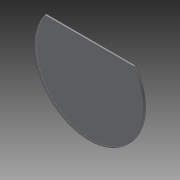
# Autodesk Inventor part: Mid Plate
Saved by Autodesk Inventor 2015 (Build 190159000, 159)
## iProperties
Created: 2014-11-13
Part Number: Mid Plate
Material: Generic
Document SubType Name: Modeling
Designer: karl
Density: 1 g/cm^3
Appearance: Default
Author: karl
Autodesk Inventor part; units mm, degrees
ref_plane "YZ Plane" through (0, 0, 0) normal (1, 0, 0) x (0, 1, 0)
ref_plane "XZ Plane" through (0, 0, 0) normal (0, 1, 0) x (-1, 0, 0)
ref_plane "XY Plane" through (0, 0, 0) normal (0, 0, 1) x (1, 0, 0)
sketch "Sketch1" plane through (0, 0, 0) normal (0, 1, 0) x (-1, 0, 0)
  circle A0 centre (0, 0) radius 90
  line L0 (73.4575, 52) -> (-73.4575, 52)
  dimension "d0" = 180
  dimension "d1" = 52
  constraints: 2 end point, 2 point on circle, 1 centre point, 1 coincident, 1 horizontal
  measures "d0" diameter of A0
  measures "d1" distance from line of point (0, 0) L0
extrude "Extrusion1" add sketch "Sketch1" along normal blind 3 contours A0 L0 picked at (17.1608, -0.9679)
sketch "Sketch2" plane through (0, 3, 0) normal (0, 1, 0) x (1, 0, 0)
  line L0 (-73.4575, -52) -> (73.4575, -52) projected
  line L1 (57, -52) -> (90, -52)
  line L2 (90, -52) -> (90, 90)
  line L3 (90, 90) -> (57, 90)
  line L4 (57, 90) -> (57, -52)
  arc A0 (73.4575, -52) -> (-73.4575, -52) centre (0, 0) ccw projected
  dimension "d4" = 57
  constraints: 8 end point, 2 parallel, 2 tangent, 1 horizontal, 1 perpendicular, 1 point on line
  measures "d4" distance from line of point (0, 0) L4
extrude "Extrusion2" cut sketch "Sketch2" against normal blind 3 contours L4 A0 L0 | L4 L3 L2 A0 | A0 L2 L1 picked at (60.2055, 26.0552)
sketch "Sketch3" plane through (0, 3, 0) normal (0, 1, 0) x (1, 0, 0)
  line L0 (29, -46) -> (-29, -46)
  line L1 (-29, -46) -> (-29, 22)
  line L2 (-29, 22) -> (29, 22)
  line L3 (29, 22) -> (29, -46)
  line L4 (-73.4575, -52) -> (57, -52) projected
  point P0 (0, 0)
  dimension "d7" = 6
  dimension "d8" = 74
  dimension "d9" = 29
  dimension "d10" = 29
  constraints: 8 end point, 2 parallel, 1 horizontal, 1 perpendicular
  measures "d7" distance between parallel lines of L4 L0
  measures "d8" distance between parallel lines of L4 L2
  measures "d9" distance from line of point (0, 0) L1
  measures "d10" distance from line of L3 point (0, 0)
extrude "Extrusion3" cut sketch "Sketch3" against normal blind 3
mirror "Mirror1" about plane through (0, 0, 0) normal (1, 0, 0) of "Extrusion2"
sketch "Sketch4" plane through (0, 3, 0) normal (0, 1, 0) x (1, 0, 0)
  line L0 (57, 69.6491) -> (57, -52) projected
  line L1 (57, -37) -> (60, -37)
  line L2 (60, -37) -> (60, -17)
  line L3 (60, -17) -> (57, -17)
  line L4 (57, -17) -> (57, -37)
  line L5 (-57, -52) -> (57, -52) projected
  line L6 (57, 13) -> (60, 13)
  line L7 (60, 13) -> (60, 33)
  line L8 (60, 33) -> (57, 33)
  line L9 (57, 33) -> (57, 13)
  point P0 (0, 0)
  dimension "d13" = 3
  dimension "d14" = 20
  dimension "d15" = 15
  dimension "d16" = 3
  dimension "d17" = 20
  dimension "d18" = 30
  constraints: 16 end point, 4 parallel, 2 horizontal, 2 perpendicular, 2 point on line
  measures "d13" distance of L3.end L2.end
  measures "d14" distance of L2.end L1.end
  measures "d15" distance between parallel lines of L5 L1
  measures "d16" distance of L8.end L7.end
  measures "d17" distance of L7.end L6.end
  measures "d18" distance between parallel lines of L3 L6
extrude "Extrusion4" add sketch "Sketch4" against normal blind 3
sketch "Sketch5" plane through (0, 3, 0) normal (0, 1, 0) x (1, 0, 0)
  line L0 (38, 53) -> (35, 53)
  line L1 (35, 53) -> (35, 43)
  line L2 (35, 43) -> (38, 43)
  line L3 (38, 43) -> (38, 53)
  line L4 (38, -42) -> (35, -42)
  line L5 (35, -42) -> (35, -32)
  line L6 (35, -32) -> (38, -32)
  line L7 (38, -32) -> (38, -42)
  line L8 (38, 8) -> (35, 8)
  line L9 (35, 8) -> (35, -12)
  line L10 (35, -12) -> (38, -12)
  line L11 (38, -12) -> (38, 8)
  line L12 (-57, -52) -> (57, -52) projected
  point P0 (0, 0)
  dimension "d21" = 3
  dimension "d22" = 10
  dimension "d23" = 3
  dimension "d24" = 10
  dimension "d25" = 3
  dimension "d26" = 20
  dimension "d27" = 10
  dimension "d28" = 20
  dimension "d29" = 35
  dimension "d30" = 35
  constraints: 24 end point, 6 parallel, 3 horizontal, 3 perpendicular, 2 point on line
  measures "d21" distance of L2.end L1.end
  measures "d22" distance of L1.end L0.end
  measures "d23" distance of L5.end L6.end
  measures "d24" distance of L4.end L5.end
  measures "d25" distance of L10.end L9.end
  measures "d26" distance of L9.end L8.end
  measures "d27" distance between parallel lines of L12 L4
  measures "d28" distance between parallel lines of L10 L6
  measures "d29" distance between parallel lines of L2 L8
  measures "d30" distance from line of point (0, 0) L5
extrude "Extrusion5" cut sketch "Sketch5" against normal blind 3
sketch "Sketch6" plane through (0, 3, 0) normal (0, 1, 0) x (1, 0, 0)
  line L0 (52.5, 31) -> (42.5, 31)
  line L1 (42.5, 31) -> (42.5, 28)
  line L2 (42.5, 28) -> (52.5, 28)
  line L3 (52.5, 28) -> (52.5, 31)
  line L4 (5, 31) -> (25, 31)
  line L5 (25, 31) -> (25, 28)
  line L6 (25, 28) -> (5, 28)
  line L7 (5, 28) -> (5, 31)
  line L8 (-57, -52) -> (57, -52) projected
  point P0 (0, 0)
  dimension "d33" = 10
  dimension "d34" = 3
  dimension "d35" = 20
  dimension "d36" = 3
  dimension "d37" = 5
  dimension "d38" = 17.5
  dimension "d39" = 80
  constraints: 16 end point, 4 parallel, 2 horizontal, 2 perpendicular, 1 point on line
  measures "d33" distance of L2.end L1.end
  measures "d34" distance of L1.end L0.end
  measures "d35" distance of L5.end L6.end
  measures "d36" distance of L4.end L5.end
  measures "d37" distance from line of point (0, 0) L7
  measures "d38" distance between parallel lines of L1 L5
  measures "d39" distance between parallel lines of L8 L6
extrude "Extrusion6" cut sketch "Sketch6" against normal blind 3
mirror "Mirror2" about plane through (0, 0, 0) normal (1, 0, 0) of "Extrusion4", "Extrusion5", "Extrusion6"
sketch "Sketch7" plane through (0, 3, 0) normal (0, 1, 0) x (1, 0, 0)
  line L0 (-1.75, 99) -> (1.75, 99)
  line L1 (1.75, 99) -> (1.75, 79)
  line L2 (1.75, 79) -> (-1.75, 79)
  line L3 (-1.75, 79) -> (-1.75, 99)
  point P0 (0, 0)
  point P1 (0, 79)
  dimension "d42" = 3.5
  dimension "d43" = 20
  dimension "d44" = 79
  constraints: 8 end point, 2 parallel, 1 horizontal, 1 midpoint, 1 perpendicular, 1 vertical alignment
  measures "d42" distance of L1.end L2.end
  measures "d43" distance of L0.end L1.end
  measures "d44" distance from line of point (0, 0) L2
extrude "Extrusion7" cut sketch "Sketch7" against normal blind 3
sketch "Sketch8" plane through (0, 3, 0) normal (0, 1, 0) x (1, 0, 0)
  line L0 (42.5, 14) -> (52.5, 14)
  line L1 (52.5, 14) -> (52.5, 11)
  line L2 (52.5, 11) -> (42.5, 11)
  line L3 (42.5, 11) -> (42.5, 14)
  line L4 (42.5, 28) -> (42.5, 31) projected
  line L5 (42.5, -37) -> (52.5, -37)
  line L6 (52.5, -37) -> (52.5, -34)
  line L7 (52.5, -34) -> (42.5, -34)
  line L8 (42.5, -34) -> (42.5, -37)
  line L9 (-57, -52) -> (57, -52) projected
  point P0 (0, 0)
  dimension "d47" = 10
  dimension "d48" = 3
  dimension "d49" = 10
  dimension "d50" = 3
  dimension "d51" = 45
  dimension "d52" = 15
  constraints: 16 end point, 4 parallel, 2 collinear, 2 horizontal, 2 perpendicular
  measures "d47" distance of L1.end L2.end
  measures "d48" distance of L0.end L1.end
  measures "d49" distance of L7.end L6.end
  measures "d50" distance of L6.end L5.end
  measures "d51" distance between parallel lines of L7 L2
  measures "d52" distance between parallel lines of L9 L5
extrude "Extrusion8" cut sketch "Sketch8" against normal blind 3
sketch "Sketch9" plane through (0, 3, 0) normal (0, 1, 0) x (1, 0, 0)
  line L0 (-57, -52) -> (57, -52) projected
  line L1 (50, -52) -> (30, -52)
  line L2 (30, -52) -> (30, -55)
  line L3 (30, -55) -> (50, -55)
  line L4 (50, -55) -> (50, -52)
  line L5 (20, -52) -> (10, -52)
  line L6 (10, -52) -> (10, -55)
  line L7 (10, -55) -> (20, -55)
  line L8 (20, -55) -> (20, -52)
  point P0 (0, 0)
  dimension "d55" = 20
  dimension "d56" = 3
  dimension "d57" = 10
  dimension "d58" = 3
  dimension "d59" = 10
  dimension "d60" = 10
  constraints: 16 end point, 4 parallel, 2 horizontal, 2 perpendicular, 2 point on line
  measures "d55" distance of L3.end L2.end
  measures "d56" distance of L2.end L1.end
  measures "d57" distance of L7.end L6.end
  measures "d58" distance of L6.end L5.end
  measures "d59" distance between parallel lines of L8 L2
  measures "d60" distance from line of point (0, 0) L6
extrude "Extrusion9" add sketch "Sketch9" against normal blind 3
sketch "Sketch10" plane through (0, 3, 0) normal (0, 1, 0) x (1, 0, 0)
  line L0 (1.75, 77) -> (4.75, 77)
  line L1 (4.75, 77) -> (4.75, 72)
  line L2 (4.75, 72) -> (1.75, 72)
  line L3 (1.75, 72) -> (1.75, 77)
  line L4 (1.75, 79) -> (-1.75, 79) projected
  line L5 (1.75, 89.983) -> (1.75, 79) projected
  point P0 (0, 0)
  dimension "d63" = 3
  dimension "d64" = 5
  dimension "d65" = 2
  constraints: 8 end point, 2 parallel, 1 collinear, 1 horizontal, 1 perpendicular
  measures "d63" distance of L1.end L2.end
  measures "d64" distance of L0.end L1.end
  measures "d65" distance between parallel lines of L4 L0
extrude "Extrusion10" cut sketch "Sketch10" against normal blind 3
mirror "Mirror3" about plane through (0, 0, 0) normal (1, 0, 0) of "Extrusion9", "Extrusion8", "Extrusion10"
sketch "Sketch11" plane through (0, 3, 0) normal (0, 1, 0) x (1, 0, 0)
  circle A0 centre (52, 48) radius 1.5
  circle A1 centre (52, 63) radius 1.5
  line L0 (57, 33) -> (57, 69.6491) projected
  line L1 (60, 33) -> (57, 33) projected
  circle A2 centre (-52, 48) radius 1.5
  circle A3 centre (-52, 63) radius 1.5
  line L2 (-57, 69.6491) -> (-57, 33) projected
  point P0 (0, 0)
  dimension "d68" = 3
  dimension "d69" = 3
  dimension "d70" = 5
  dimension "d71" = 15
  dimension "d72" = 15
  dimension "d73" = 3
  dimension "d74" = 3
  dimension "d75" = 5
  constraints: 4 centre point, 2 horizontal alignment, 2 vertical alignment
  measures "d68" diameter of A0
  measures "d69" diameter of A1
  measures "d70" distance from line of L0 A0.centre
  measures "d71" distance of A1.centre A0.centre
  measures "d72" distance from line of L1 A0.centre
  measures "d73" diameter of A2
  measures "d74" diameter of A3
  measures "d75" distance from line of L2 A2.centre
extrude "Extrusion11" cut sketch "Sketch11" against normal blind 3
equation "\"d10\" = d9"
body "Solid1"
